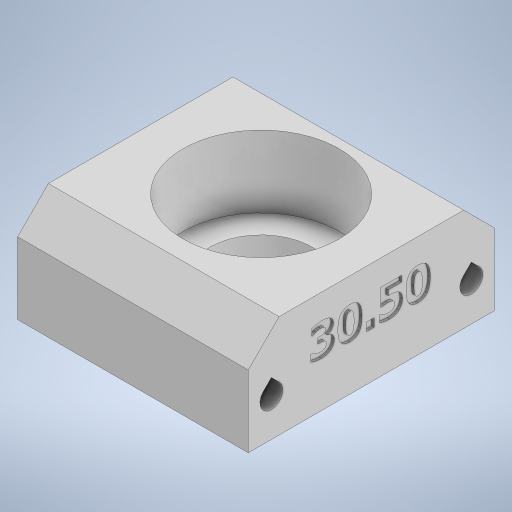
# Autodesk Inventor part: Część1-02
Saved by Autodesk Inventor 2023 (Build 270158000, 158)
## iProperties
Created: 2023-04-06
Part Number: Część1-02
Material: Ogólny
Document SubType Name: Modeling
Designer: Kamil
Density: 1 g/cm^3
Appearance: Domyślna
Author: Kamil
Autodesk Inventor part; units mm, degrees
ref_plane "YZ Plane" through (0, 0, 0) normal (1, 0, 0) x (0, 1, 0)
ref_plane "XZ Plane" through (0, 0, 0) normal (0, 1, 0) x (-1, 0, 0)
ref_plane "XY Plane" through (0, 0, 0) normal (0, 0, 1) x (1, 0, 0)
sketch "Szkic1" plane through (0, 0, 0) normal (0, 1, 0) x (-1, 0, 0)
  line L0 (22.5, 24) -> (-22.5, 24)
  line L1 (-22.5, 24) -> (-22.5, -24)
  line L2 (-22.5, -24) -> (22.5, -24)
  line L3 (22.5, -24) -> (22.5, 24)
  line L4 (22.5, 24) -> (-22.5, -24) construction
  line L5 (-22.5, 24) -> (22.5, -24) construction
  point P0 (0, 0)
  dimension "d0" = 45
  dimension "d1" = 48
  constraints: 12 end point, 2 midpoint, 2 parallel, 1 horizontal, 1 perpendicular
  measures "d0" distance of L2.end L1.end
  measures "d1" distance of L1.end L0.end
extrude "Wyciągnięcie proste1" add sketch "Szkic1" along normal blind 20
sketch "Szkic2" plane through (0, 20, 0) normal (0, 1, 0) x (1, 0, 0)
  line L0 (0, 0) -> (0, 1) construction
  dimension "d4" = 1
  constraints: 2 end point, 1 coincident, 1 vertical
  measures "d4" distance of L0.start L0.end
hole "Otwór1" at (0, 20, -1) direction (0, -1, 0) diameter 20 end through all counterbore diameter 30.5 counterbore depth 14
chamfer "Faza1" distance 6 angle 45 2 edges at (0, 20, -24) (0, 20, 24)
sketch "Szkic3" plane through (22.5, 0, 24) normal (1, 0, 0) x (0, 0, -1)
  line L0 (0, 0) -> (4.5, 0)
  line L1 (24, 0) -> (24, 9.8003)
  arc A0 (2.909, 8.891) -> (6.091, 8.891) centre (4.5, 7.3) ccw
  line L2 (4.5, 10.482) -> (6.091, 8.891)
  line L3 (4.5, 10.482) -> (2.909, 8.891)
  line L4 (0, 0) -> (48, 0) projected
  line L5 (0, 0) -> (0, 14) projected
  arc A1 (41.909, 8.891) -> (45.091, 8.891) centre (43.5, 7.3) ccw
  line L6 (43.5, 10.482) -> (41.909, 8.891)
  line L7 (43.5, 10.482) -> (45.091, 8.891)
  dimension "d17" = 4.5
  dimension "d20" = 7.3
  dimension "d21" = 4.5
  constraints: 12 end point, 4 point on circle, 4 symmetric about line, 2 centre point, 2 coincident, 1 horizontal, 1 tangent, 1 vertical, 1 other
  measures "d17" diameter of A0
  measures "d20" distance from line of L4 A0.centre
  measures "d21" distance from line of L5 A0.centre
extrude "Wyciągnięcie proste2" cut sketch "Szkic3" against normal through all
sketch "Szkic4" plane through (22.5, 0, -24) normal (0, 0, -1) x (-1, 0, 0)
  line L0 (13, 10) -> (32, 10) construction
  line L1 (32, 10) -> (32, 4) construction
  line L2 (32, 4) -> (13, 4) construction
  line L3 (13, 4) -> (13, 10) construction
  line L4 (22.5, -0.0035) -> (22.5, 22.4866) construction
  line L5 (0, 8.891) -> (45, 8.891) construction
  line L6 (0, 0) -> (0, 14) construction
  line L7 (17.8296, 3.7764) -> (13.8008, 3.7764)
  line L8 (13.8008, 3.7764) -> (13.8008, 4.8392)
  line L9 (13.8008, 4.8392) -> (15.0861, 4.8392)
  line L10 (15.0861, 4.8392) -> (15.0861, 8.0672)
  line L11 (15.0861, 8.0672) -> (13.8008, 8.0672)
  line L12 (13.8008, 8.0672) -> (13.8008, 9.0608)
  spline S0 degree 2 poles (13.8008, 9.0608) (14.0826, 9.0608) (14.6412, 9.1349) (14.8092, 9.214) knots 0 0 0 1 2 2 2
  spline S1 degree 2 poles (14.8092, 9.214) (15.002, 9.3129) (15.2195, 9.6441) (15.2393, 9.8912) knots 0 0 0 1 2 2 2
  line L13 (15.2393, 9.8912) -> (16.574, 9.8912)
  line L14 (16.574, 9.8912) -> (16.574, 4.8392)
  line L15 (16.574, 4.8392) -> (17.8296, 4.8392)
  line L16 (17.8296, 4.8392) -> (17.8296, 3.7764)
  line L17 (20.3754, 3.7764) -> (18.927, 3.7764)
  line L18 (18.927, 3.7764) -> (18.927, 5.3879)
  line L19 (18.927, 5.3879) -> (20.3754, 5.3879)
  line L20 (20.3754, 5.3879) -> (20.3754, 3.7764)
  spline S2 degree 2 poles (25.986, 6.8264) (25.986, 6.0355) (25.7339, 4.8491) (25.4521, 4.4487) knots 0 0 0 1 2 2 2
  spline S3 degree 2 poles (25.4521, 4.4487) (25.1753, 4.0532) (24.2806, 3.6479) (23.6379, 3.6479) knots 0 0 0 1 2 2 2
  spline S4 degree 2 poles (23.6379, 3.6479) (22.9904, 3.6479) (22.1006, 4.0532) (21.8188, 4.4586) knots 0 0 0 1 2 2 2
  spline S5 degree 2 poles (21.8188, 4.4586) (21.537, 4.859) (21.2849, 6.0355) (21.2849, 6.8264) knots 0 0 0 1 2 2 2
  spline S6 degree 2 poles (21.2849, 6.8264) (21.2849, 7.6371) (21.537, 8.784) (21.8237, 9.1992) knots 0 0 0 1 2 2 2
  spline S7 degree 2 poles (21.8237, 9.1992) (22.1105, 9.6045) (23.0151, 10) (23.6379, 10) knots 0 0 0 1 2 2 2
  spline S8 degree 2 poles (23.6379, 10) (24.2954, 10) (25.1753, 9.5848) (25.4571, 9.1745) knots 0 0 0 1 2 2 2
  spline S9 degree 2 poles (25.4571, 9.1745) (25.7339, 8.7741) (25.986, 7.5926) (25.986, 6.8264) knots 0 0 0 1 2 2 2
  spline S10 degree 2 poles (24.4486, 6.8264) (24.4486, 7.9584) (24.0779, 8.8729) (23.6379, 8.8729) knots 0 0 0 1 2 2 2
  spline S11 degree 2 poles (23.6379, 8.8729) (23.198, 8.8729) (22.8223, 7.9584) (22.8223, 6.8215) knots 0 0 0 1 2 2 2
  spline S12 degree 2 poles (22.8223, 6.8215) (22.8223, 5.7043) (23.198, 4.775) (23.6379, 4.775) knots 0 0 0 1 2 2 2
  spline S13 degree 2 poles (23.6379, 4.775) (24.0729, 4.775) (24.4486, 5.7043) (24.4486, 6.8264) knots 0 0 0 1 2 2 2
  spline S14 degree 2 poles (31.3297, 6.8264) (31.3297, 6.0355) (31.0776, 4.8491) (30.7958, 4.4487) knots 0 0 0 1 2 2 2
  spline S15 degree 2 poles (30.7958, 4.4487) (30.519, 4.0532) (29.6242, 3.6479) (28.9816, 3.6479) knots 0 0 0 1 2 2 2
  spline S16 degree 2 poles (28.9816, 3.6479) (28.334, 3.6479) (27.4442, 4.0532) (27.1625, 4.4586) knots 0 0 0 1 2 2 2
  spline S17 degree 2 poles (27.1625, 4.4586) (26.8807, 4.859) (26.6286, 6.0355) (26.6286, 6.8264) knots 0 0 0 1 2 2 2
  spline S18 degree 2 poles (26.6286, 6.8264) (26.6286, 7.6371) (26.8807, 8.784) (27.1674, 9.1992) knots 0 0 0 1 2 2 2
  spline S19 degree 2 poles (27.1674, 9.1992) (27.4541, 9.6045) (28.3588, 10) (28.9816, 10) knots 0 0 0 1 2 2 2
  spline S20 degree 2 poles (28.9816, 10) (29.6391, 10) (30.519, 9.5848) (30.8007, 9.1745) knots 0 0 0 1 2 2 2
  spline S21 degree 2 poles (30.8007, 9.1745) (31.0776, 8.7741) (31.3297, 7.5926) (31.3297, 6.8264) knots 0 0 0 1 2 2 2
  spline S22 degree 2 poles (29.7923, 6.8264) (29.7923, 7.9584) (29.4216, 8.8729) (28.9816, 8.8729) knots 0 0 0 1 2 2 2
  spline S23 degree 2 poles (28.9816, 8.8729) (28.5417, 8.8729) (28.166, 7.9584) (28.166, 6.8215) knots 0 0 0 1 2 2 2
  spline S24 degree 2 poles (28.166, 6.8215) (28.166, 5.7043) (28.5417, 4.775) (28.9816, 4.775) knots 0 0 0 1 2 2 2
  spline S25 degree 2 poles (28.9816, 4.775) (29.4166, 4.775) (29.7923, 5.7043) (29.7923, 6.8264) knots 0 0 0 1 2 2 2
  point P0 (22.5, 0)
  point P1 (22.5, 10)
  point P2 (22.5, 8.891)
  point P3 (32, 7)
  point P4 (0, 7)
  dimension "d4" = 1
  constraints: 4 midpoint, 2 end point, 1 horizontal alignment, 1 point on line, 1 vertical, 1 vertical alignment, 2 other
extrude "Wyciągnięcie proste3" cut sketch "Szkic4" against normal blind 0.5
sketch "Szkic5" plane through (22.5, 0, 24) normal (1, 0, 0) x (0, 0, -1)
  line L0 (11.8023, 15.1728) -> (36.4562, 15.1728) construction
  line L1 (36.4562, 15.1728) -> (36.4562, 8.8157) construction
  line L2 (36.4562, 8.8157) -> (11.8023, 8.8157) construction
  line L3 (11.8023, 8.8157) -> (11.8023, 15.1728) construction
  spline S0 degree 2 poles (16.7505, 10.793) (16.7505, 10.3432) (16.4193, 9.6066) (16.098, 9.3496) knots 0 0 0 1 2 2 2
  spline S1 degree 2 poles (16.098, 9.3496) (15.7767, 9.0925) (14.9017, 8.8157) (14.2739, 8.8157) knots 0 0 0 1 2 2 2
  spline S2 degree 2 poles (14.2739, 8.8157) (13.5621, 8.8157) (12.5438, 9.053) (12.2225, 9.2013) knots 0 0 0 1 2 2 2
  line L4 (12.2225, 9.2013) -> (12.2225, 10.5261)
  line L5 (12.2225, 10.5261) -> (12.3708, 10.5261)
  spline S3 degree 2 poles (12.3708, 10.5261) (12.7069, 10.3135) (13.6115, 9.9972) (13.9872, 9.9972) knots 0 0 0 1 2 2 2
  spline S4 degree 2 poles (13.9872, 9.9972) (14.2097, 9.9972) (14.7287, 10.0762) (14.9067, 10.2048) knots 0 0 0 1 2 2 2
  spline S5 degree 2 poles (14.9067, 10.2048) (15.0451, 10.3086) (15.2132, 10.6101) (15.2132, 10.882) knots 0 0 0 1 2 2 2
  spline S6 degree 2 poles (15.2132, 10.882) (15.2132, 11.1539) (14.9759, 11.4455) (14.7781, 11.5147) knots 0 0 0 1 2 2 2
  spline S7 degree 2 poles (14.7781, 11.5147) (14.5804, 11.5839) (14.0317, 11.5988) (13.8191, 11.5988) knots 0 0 0 1 2 2 2
  line L6 (13.8191, 11.5988) -> (13.5572, 11.5988)
  line L7 (13.5572, 11.5988) -> (13.5572, 12.6715)
  line L8 (13.5572, 12.6715) -> (13.7994, 12.6715)
  spline S8 degree 2 poles (13.7994, 12.6715) (14.0762, 12.6715) (14.5458, 12.7209) (14.7089, 12.795) knots 0 0 0 1 2 2 2
  spline S9 degree 2 poles (14.7089, 12.795) (14.8721, 12.8741) (15.055, 13.151) (15.055, 13.3882) knots 0 0 0 1 2 2 2
  spline S10 degree 2 poles (15.055, 13.3882) (15.055, 13.5761) (14.882, 13.8084) (14.7584, 13.8727) knots 0 0 0 1 2 2 2
  spline S11 degree 2 poles (14.7584, 13.8727) (14.6101, 13.9468) (14.2146, 13.9963) (14.0762, 13.9963) knots 0 0 0 1 2 2 2
  spline S12 degree 2 poles (14.0762, 13.9963) (13.8537, 13.9963) (13.3841, 13.8925) (13.1666, 13.8084) knots 0 0 0 1 2 2 2
  spline S13 degree 2 poles (13.1666, 13.8084) (12.9936, 13.7442) (12.6179, 13.5365) (12.529, 13.4822) knots 0 0 0 1 2 2 2
  line L9 (12.529, 13.4822) -> (12.4004, 13.4822)
  line L10 (12.4004, 13.4822) -> (12.4004, 14.7872)
  spline S14 degree 2 poles (12.4004, 14.7872) (12.7168, 14.9207) (13.7845, 15.1728) (14.3431, 15.1728) knots 0 0 0 1 2 2 2
  spline S15 degree 2 poles (14.3431, 15.1728) (14.8869, 15.1728) (15.6877, 14.9849) (15.9695, 14.802) knots 0 0 0 1 2 2 2
  spline S16 degree 2 poles (15.9695, 14.802) (16.2809, 14.6092) (16.5923, 14.016) (16.5923, 13.6453) knots 0 0 0 1 2 2 2
  spline S17 degree 2 poles (16.5923, 13.6453) (16.5923, 13.1213) (15.9892, 12.3403) (15.4949, 12.2266) knots 0 0 0 1 2 2 2
  line L11 (15.4949, 12.2266) -> (15.4949, 12.1672)
  spline S18 degree 2 poles (15.4949, 12.1672) (15.7124, 12.1376) (16.1277, 11.9794) (16.3254, 11.8014) knots 0 0 0 1 2 2 2
  spline S19 degree 2 poles (16.3254, 11.8014) (16.5083, 11.6433) (16.7505, 11.139) (16.7505, 10.793) knots 0 0 0 1 2 2 2
  spline S20 degree 2 poles (22.1683, 11.9942) (22.1683, 11.2033) (21.9162, 10.0169) (21.6345, 9.6165) knots 0 0 0 1 2 2 2
  spline S21 degree 2 poles (21.6345, 9.6165) (21.3576, 9.2211) (20.4629, 8.8157) (19.8203, 8.8157) knots 0 0 0 1 2 2 2
  spline S22 degree 2 poles (19.8203, 8.8157) (19.1727, 8.8157) (18.2829, 9.2211) (18.0012, 9.6264) knots 0 0 0 1 2 2 2
  spline S23 degree 2 poles (18.0012, 9.6264) (17.7194, 10.0268) (17.4673, 11.2033) (17.4673, 11.9942) knots 0 0 0 1 2 2 2
  spline S24 degree 2 poles (17.4673, 11.9942) (17.4673, 12.8049) (17.7194, 13.9518) (18.0061, 14.367) knots 0 0 0 1 2 2 2
  spline S25 degree 2 poles (18.0061, 14.367) (18.2928, 14.7724) (19.1974, 15.1678) (19.8203, 15.1678) knots 0 0 0 1 2 2 2
  spline S26 degree 2 poles (19.8203, 15.1678) (20.4777, 15.1678) (21.3576, 14.7526) (21.6394, 14.3423) knots 0 0 0 1 2 2 2
  spline S27 degree 2 poles (21.6394, 14.3423) (21.9162, 13.9419) (22.1683, 12.7604) (22.1683, 11.9942) knots 0 0 0 1 2 2 2
  spline S28 degree 2 poles (20.631, 11.9942) (20.631, 13.1262) (20.2602, 14.0407) (19.8203, 14.0407) knots 0 0 0 1 2 2 2
  spline S29 degree 2 poles (19.8203, 14.0407) (19.3803, 14.0407) (19.0046, 13.1262) (19.0046, 11.9893) knots 0 0 0 1 2 2 2
  spline S30 degree 2 poles (19.0046, 11.9893) (19.0046, 10.8721) (19.3803, 9.9428) (19.8203, 9.9428) knots 0 0 0 1 2 2 2
  spline S31 degree 2 poles (19.8203, 9.9428) (20.2553, 9.9428) (20.631, 10.8721) (20.631, 11.9942) knots 0 0 0 1 2 2 2
  line L12 (24.5213, 8.9442) -> (23.073, 8.9442)
  line L13 (23.073, 8.9442) -> (23.073, 10.5557)
  line L14 (23.073, 10.5557) -> (24.5213, 10.5557)
  line L15 (24.5213, 10.5557) -> (24.5213, 8.9442)
  spline S32 degree 2 poles (30.0726, 11.0105) (30.0726, 10.531) (29.7464, 9.7203) (29.4251, 9.4287) knots 0 0 0 1 2 2 2
  spline S33 degree 2 poles (29.4251, 9.4287) (29.1038, 9.137) (28.2238, 8.8157) (27.5812, 8.8157) knots 0 0 0 1 2 2 2
  spline S34 degree 2 poles (27.5812, 8.8157) (26.899, 8.8207) (25.9203, 9.0431) (25.599, 9.1865) knots 0 0 0 1 2 2 2
  line L16 (25.599, 9.1865) -> (25.599, 10.5162)
  line L17 (25.599, 10.5162) -> (25.7374, 10.5162)
  spline S35 degree 2 poles (25.7374, 10.5162) (25.856, 10.4519) (26.1427, 10.2839) (26.3751, 10.1949) knots 0 0 0 1 2 2 2
  spline S36 degree 2 poles (26.3751, 10.1949) (26.5926, 10.1108) (27.0424, 9.9972) (27.3143, 9.9972) knots 0 0 0 1 2 2 2
  spline S37 degree 2 poles (27.3143, 9.9972) (27.5516, 9.9972) (28.1052, 10.1158) (28.2733, 10.274) knots 0 0 0 1 2 2 2
  spline S38 degree 2 poles (28.2733, 10.274) (28.3969, 10.3976) (28.5353, 10.6991) (28.5353, 10.9512) knots 0 0 0 1 2 2 2
  spline S39 degree 2 poles (28.5353, 10.9512) (28.5353, 11.1687) (28.3573, 11.4752) (28.214, 11.5691) knots 0 0 0 1 2 2 2
  spline S40 degree 2 poles (28.214, 11.5691) (28.0063, 11.7075) (27.4132, 11.7866) (27.2006, 11.7866) knots 0 0 0 1 2 2 2
  spline S41 degree 2 poles (27.2006, 11.7866) (26.8644, 11.7866) (26.2268, 11.6779) (25.9944, 11.6185) knots 0 0 0 1 2 2 2
  line L18 (25.9944, 11.6185) -> (25.861, 11.6185)
  line L19 (25.861, 11.6185) -> (25.861, 15.0442)
  line L20 (25.861, 15.0442) -> (29.9046, 15.0442)
  line L21 (29.9046, 15.0442) -> (29.9046, 13.8925)
  line L22 (29.9046, 13.8925) -> (27.3093, 13.8925)
  line L23 (27.3093, 13.8925) -> (27.3093, 12.8791)
  spline S42 degree 2 poles (27.3093, 12.8791) (27.4329, 12.889) (27.774, 12.8989) (27.8679, 12.8989) knots 0 0 0 1 2 2 2
  spline S43 degree 2 poles (27.8679, 12.8989) (28.3079, 12.8989) (29.0494, 12.7209) (29.341, 12.538) knots 0 0 0 1 2 2 2
  spline S44 degree 2 poles (29.341, 12.538) (29.6871, 12.3106) (30.0726, 11.5543) (30.0726, 11.0105) knots 0 0 0 1 2 2 2
  spline S45 degree 2 poles (35.4756, 11.9942) (35.4756, 11.2033) (35.2235, 10.0169) (34.9418, 9.6165) knots 0 0 0 1 2 2 2
  spline S46 degree 2 poles (34.9418, 9.6165) (34.6649, 9.2211) (33.7702, 8.8157) (33.1276, 8.8157) knots 0 0 0 1 2 2 2
  spline S47 degree 2 poles (33.1276, 8.8157) (32.48, 8.8157) (31.5902, 9.2211) (31.3085, 9.6264) knots 0 0 0 1 2 2 2
  spline S48 degree 2 poles (31.3085, 9.6264) (31.0267, 10.0268) (30.7746, 11.2033) (30.7746, 11.9942) knots 0 0 0 1 2 2 2
  spline S49 degree 2 poles (30.7746, 11.9942) (30.7746, 12.8049) (31.0267, 13.9518) (31.3134, 14.367) knots 0 0 0 1 2 2 2
  spline S50 degree 2 poles (31.3134, 14.367) (31.6001, 14.7724) (32.5047, 15.1678) (33.1276, 15.1678) knots 0 0 0 1 2 2 2
  spline S51 degree 2 poles (33.1276, 15.1678) (33.785, 15.1678) (34.6649, 14.7526) (34.9467, 14.3423) knots 0 0 0 1 2 2 2
  spline S52 degree 2 poles (34.9467, 14.3423) (35.2235, 13.9419) (35.4756, 12.7604) (35.4756, 11.9942) knots 0 0 0 1 2 2 2
  spline S53 degree 2 poles (33.9383, 11.9942) (33.9383, 13.1262) (33.5675, 14.0407) (33.1276, 14.0407) knots 0 0 0 1 2 2 2
  spline S54 degree 2 poles (33.1276, 14.0407) (32.6876, 14.0407) (32.3119, 13.1262) (32.3119, 11.9893) knots 0 0 0 1 2 2 2
  spline S55 degree 2 poles (32.3119, 11.9893) (32.3119, 10.8721) (32.6876, 9.9428) (33.1276, 9.9428) knots 0 0 0 1 2 2 2
  spline S56 degree 2 poles (33.1276, 9.9428) (33.5626, 9.9428) (33.9383, 10.8721) (33.9383, 11.9942) knots 0 0 0 1 2 2 2
  point P0 (24, 0)
  dimension "srednica_lozyska" = 30.5
  constraints: 2 other
extrude "Wyciągnięcie proste4" cut sketch "Szkic5" against normal blind 0.5
